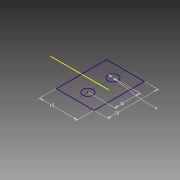
# Autodesk Inventor part: Belt Clamp
Saved by Autodesk Inventor 2015 (Build 190159000, 159)
## iProperties
Created: 2015-05-14
Part Number: Belt Clamp
Material: Generic
Document SubType Name: Modeling
Designer: pltwe4
Density: 1 g/cm^3
Appearance: Default
Author: pltwe4
Autodesk Inventor part; units mm, degrees
ref_plane "YZ Plane" through (0, 0, 0) normal (1, 0, 0) x (0, 1, 0)
ref_plane "XZ Plane" through (0, 0, 0) normal (0, 1, 0) x (-1, 0, 0)
ref_plane "XY Plane" through (0, 0, 0) normal (0, 0, 1) x (1, 0, 0)
sketch "Sketch1" plane through (0, 0, 0) normal (0, 0, 1) x (1, 0, 0)
  circle A0 centre (0, 10) radius 2
  circle A1 centre (0, -10) radius 2
  line L0 (7.5, 15) -> (-7.5, 15)
  line L1 (-7.5, 15) -> (-7.5, -15)
  line L2 (-7.5, -15) -> (7.5, -15)
  line L3 (7.5, -15) -> (7.5, 15)
  line L4 (-10.5, 0) -> (10.5, 0) projected
  line L5 (0, 15) -> (0, -15) construction
  point P0 (0, 0)
  dimension "d0" = 4
  dimension "d1" = 15
  dimension "d2" = 30
  dimension "d3" = 20
  constraints: 10 end point, 3 midpoint, 2 centre point, 2 parallel, 1 horizontal, 1 perpendicular, 1 point on line, 2 other
  measures "d0" diameter of A0
  measures "d1" distance between parallel lines of L1 L3
  measures "d2" distance of L2.end L0.start
  measures "d3" distance of A1.centre A0.centre
extrude "Extrusion1" add sketch "Sketch1" along normal blind 4
sketch "Sketch2" plane through (0, 0, 4) normal (0, 0, 1) x (1, 0, 0)
  circle A0 centre (0, -10) radius 2 projected
  circle A1 centre (0, 10) radius 2 projected
  line L0 (7.5, 15) -> (-7.5, 15) projected
  line L1 (-7.5, 15) -> (-7.5, -15) projected
  line L2 (-7.5, -15) -> (7.5, -15) projected
  line L3 (7.5, -15) -> (7.5, 15) projected
  line L4 (7.5, -15) -> (7.5, 15) projected
  line L5 (-7.5, -5) -> (7.5, -5)
  line L6 (7.5, -5) -> (7.5, 5)
  line L7 (7.5, 5) -> (-7.5, 5)
  line L8 (-7.5, 5) -> (-7.5, -5)
  line L9 (-7.5, -5) -> (7.5, 5) construction
  line L10 (7.5, -5) -> (-7.5, 5) construction
  point P0 (0, 0)
  dimension "d6" = 10
  constraints: 12 end point, 2 midpoint, 2 parallel, 1 horizontal, 1 perpendicular, 1 point on line
  measures "d6" distance between parallel lines of L5 L7
extrude "Extrusion2" add sketch "Sketch2" along normal blind 12.262 contours L3 L5 L1 L7
sketch "Sketch3" plane through (-7.5, -5, 4) normal (0, -1, 0) x (1, 0, 0)
  line L0 (15, 0) -> (0, 0) projected
  line L1 (15, 0) -> (15, 12.262) projected
  line L2 (0, 12.262) -> (15, 12.262) projected
  line L3 (0, 0) -> (0, 12.262) projected
  line L4 (0, -4) -> (15, -4) projected
  line L5 (15, -4) -> (15, 0) projected
  line L6 (0, 0) -> (15, 0) projected
  line L7 (0, -4) -> (0, 0) projected
  line L8 (0, 9.262) -> (15, 9.262)
  line L9 (0, 0) -> (0, 12.262) projected
  arc A0 (0.4989, 10.3302) -> (0, 9.532) centre (0, 10.087) ccw
  arc A1 (2, 9.532) -> (1.5011, 10.3302) centre (2, 10.087) ccw
  line L10 (0.7402, 9.892) -> (1.2598, 9.892)
  line L11 (0, 9.532) -> (2, 9.532) construction
  line L12 (0, 10.642) -> (2, 10.642) construction
  arc A2 (0.5915, 10.0224) -> (0.4989, 10.3302) centre (-0.4, 9.892) ccw
  arc A3 (1.5011, 10.3302) -> (1.4085, 10.0224) centre (2.4, 9.892) ccw
  line L13 (2, 9.532) -> (2, 9.262)
  line L14 (0, 9.532) -> (0, 9.262)
  line L15 (2, 9.532) -> (2, 10.642)
  line L16 (0, 10.642) -> (0, 9.532)
  arc A4 (0.5915, 10.0224) -> (0.7402, 9.892) centre (0.7402, 10.042) ccw
  arc A5 (1.2598, 9.892) -> (1.4085, 10.0224) centre (1.2598, 10.042) ccw
  point P0 (7.5, -4)
  dimension "d9" = 13.262
  dimension "d10" = 2
  dimension "d11" = 1.11
  dimension "d16" = 1.38
  dimension "d17" = 0.75
  dimension "d18" = 2
  dimension "d19" = 0.4
  dimension "d21" = 0.4
  dimension "d22" = 1
  dimension "d23" = 0.3
  constraints: 16 end point, 14 point on circle, 8 point on line, 6 centre point, 6 tangent, 3 horizontal, 2 collinear, 2 equal radius, 1 parallel, 1 perpendicular
  measures "d9" distance between parallel lines of L4 L8
  measures "d10" distance of A0.centre A1.centre
  measures "d11" diameter of A1
  measures "d16" distance between parallel lines of L8 L12
  measures "d17" distance between parallel lines of L12 L10
  measures "d18" diameter of A2
  measures "d19" horizontal distance of A2.centre A0.centre
  measures "d21" horizontal distance of A3.centre A1.centre
  measures "d22" radius of A3
  measures "d23" diameter of A4
extrude "Extrusion3" cut sketch "Sketch3" against normal blind 8 contours L3 A0 A2 A4 L10 A5 A3 A1 L15 L13 L8
pattern_linear "Rectangular Pattern1" count 8 spacing 2 along (1, 0, 0) of "Extrusion3"
body "Solid1"
